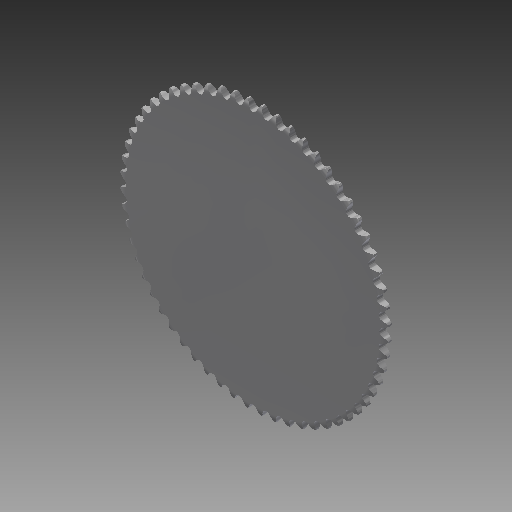
# Autodesk Inventor part: Roller Chain Sprocket2
Saved by Autodesk Inventor 2018.2 (Build 222227000, 227)
## iProperties
Created: 2018-02-09
Part Number: Roller Chain Sprocket2
Material: Steel
Document SubType Name: Modeling
Designer: steele
Density: 1 g/cm^3
Appearance: Steel
CustomPartVersion: 1
Author: steele
Autodesk Inventor part; units mm, degrees
ref_plane "YZ Plane" through (0, 0, 0) normal (1, 0, 0) x (0, 1, 0)
ref_plane "XZ Plane" through (0, 0, 0) normal (0, 1, 0) x (-1, 0, 0)
ref_plane "XY Plane" through (0, 0, 0) normal (0, 0, 1) x (1, 0, 0)
sketch "Theoretical Tooth Profile" plane through (0, 0, 0) normal (0, 0, 1) x (1, 0, 0)
  circle A0 centre (0, 0) radius 90.9986 construction
  line L0 (0, 0) -> (0, 90.9986) construction
  line L1 (0, 0) -> (9.5119, 90.5001) construction
  circle A1 centre (0, 0) radius 93.7314
  arc A2 (-2.096, 89.4758) -> (2.096, 89.4758) centre (0, 90.9986) ccw
  line L2 (0, 90.9986) -> (9.5119, 90.5001) construction
  line L3 (0, 90.9986) -> (3.2878, 93.3874) construction
  line L4 (3.2878, 93.3874) -> (-3.0069, 91.2281) construction
  arc A3 (4.3573, 93.6301) -> (3.2534, 91.9467) centre (7.1023, 90.6264) ccw
  arc A4 (-3.2534, 91.9467) -> (-4.3573, 93.6301) centre (-7.1023, 90.6264) ccw
  line L5 (-7.1023, 90.6264) -> (-3.2534, 91.9467) construction
  arc A5 (-3.0069, 91.2281) -> (-2.096, 89.4758) centre (3.2878, 93.3874) ccw
  line L6 (-3.0069, 91.2281) -> (-3.2534, 91.9467)
  arc A6 (2.096, 89.4758) -> (3.0069, 91.2281) centre (-3.2878, 93.3874) ccw
  line L7 (3.2534, 91.9467) -> (3.0069, 91.2281)
  line L8 (0, 0) -> (4.9055, 93.603) construction
  point P0 (4.756, 90.7494)
  dimension "d0" = 181.9973
  dimension "d2" = 6
  dimension "d3" = 2.5908
  dimension "d10" = 126
  dimension "d11" = 17.067
  dimension "d12" = 4.064
  dimension "d13" = 6.6548
  dimension "d14" = 7.112
  dimension "d23" = 2.8575
  constraints: 18 end point, 15 point on circle, 7 centre point, 3 coincident, 3 point on line, 3 symmetric about line, 3 tangent, 1 equal radius, 1 midpoint, 1 parallel, 1 vertical, 1 other
  measures "d0" diameter of A0
  measures "d2" angle of L1 L0
  measures "d3" radius of A2
  measures "d10" angle of L3 L0
  measures "d11" angle of L4 L3
  measures "d12" distance of L2.start L3.end
  measures "d13" distance of L3.end L4.end
  measures "d14" distance of A3.centre L0.end
  measures "d23" distance from line of L8.end L2
sketch "Tooth Profile" plane through (0, 0, 0) normal (0, 0, 1) x (1, 0, 0)
  circle A0 centre (0, 0) radius 93.7314 projected
  line L0 (0, 0) -> (0, 90.9986) construction
  line L1 (0, 90.9986) -> (2.4227, 90.0807) construction
  arc A1 (-2.4227, 90.0807) -> (2.4227, 90.0807) centre (0, 90.9986) ccw
  line L2 (-2.4227, 90.0807) -> (0, 90.9986) construction
  arc A2 (-2.4227, 90.0807) -> (-3.9883, 93.6465) centre (-37.7664, 76.6902) ccw
  arc A3 (3.9883, 93.6465) -> (2.4227, 90.0807) centre (37.7664, 76.6902) ccw
  dimension "d44" = 138.5
  dimension "d45" = 2.5908
  dimension "d46" = 37.7952
  constraints: 8 point on circle, 7 end point, 3 centre point, 2 tangent, 1 coincident, 1 equal radius, 1 symmetric about line, 1 vertical
  measures "d44" angle of L1 L2
  measures "d45" radius of A1
  measures "d46" radius of A3
sketch "Section Profile" plane through (0, 0, 0) normal (1, 0, 0) x (0, 1, 0)
  line L0 (93.7314, 0) -> (-93.7314, 0) projected
  line L1 (85.3494, 2.2967) -> (-85.3494, 2.2967)
  line L2 (-85.3494, 2.2967) -> (-85.3494, -2.2967)
  line L3 (-85.3494, -2.2967) -> (85.3494, -2.2967)
  line L4 (85.3494, -2.2967) -> (85.3494, 2.2967)
  line L5 (85.3494, 2.2967) -> (93.7314, 2.2967) construction
  line L6 (93.7314, 2.2967) -> (93.7314, -2.2967) construction
  line L7 (93.7314, -2.2967) -> (85.3494, -2.2967) construction
  line L8 (85.3494, -2.2967) -> (85.3494, 2.2967)
  arc A0 (93.7314, 1.106) -> (88.9677, 2.2967) centre (88.9677, -7.8284) ccw
  arc A1 (88.9677, -2.2967) -> (93.7314, -1.106) centre (88.9677, 7.8284) ccw
  line L9 (88.9677, 2.2967) -> (0, 2.2967)
  line L10 (0, 2.2967) -> (0, -2.2967)
  line L11 (0, -2.2967) -> (88.9677, -2.2967)
  line L12 (0, 2.2967) -> (0, -2.2967)
  line L13 (93.7314, 1.106) -> (93.7314, -1.106)
  point P0 (0, 0)
  point P1 (0, 0)
  dimension "d30" = 4.5933
  dimension "d31" = 170.6988
  dimension "d32" = 4.5933
  dimension "d33" = 1.1906
  dimension "d34" = 10.1251
  dimension "d43" = 2.2967
  constraints: 26 end point, 7 midpoint, 5 perpendicular, 4 parallel, 4 point on circle, 3 point on line, 3 symmetric about line, 2 centre point, 2 horizontal, 2 tangent, 1 collinear, 1 other
  measures "d30" distance between parallel lines of L7 L5
  measures "d31" distance between parallel lines of L2 L4
  measures "d32" distance between parallel lines of L3 L1
  measures "d33" distance from line of L13.start L5
  measures "d34" radius of A0
  measures "d43" distance between parallel lines of L3 L0
revolve "Shroud" add sketch "Section Profile" angle 360 about axis through (0, 0, 2.2967) along (0, 0, -1) contours L10 L3 L2 L0 | L0 L2 L1 L10
revolve "Strand" add sketch "Section Profile" angle 360 about axis through (0, 0, 2.2967) along (0, 0, -1) contours L13 A1 L11 L4 L0 | L0 L4 L9 A0 L13 | L4 L3 L10 L0 | L0 L10 L1 L4
pattern_of_one "Strand Pattern"
extrude "Theoretical Tooth" cut sketch "Theoretical Tooth Profile" along normal through all both and the other way through all contours A3 L7 A6 A2 A5 L6 A4 A1 picked at (0.4843, 91.2592)
extrude "Tooth" [suppressed]
pattern_circular "Tooth Pattern" count 60 over 360 about axis through (0, 0, -10) along (0, 0, 1) of "Theoretical Tooth"
ref_plane "Timing Plane" through (0, 90.9986, 0) normal (1, 0, 0) x (0, 1, 0)
equation "\"d3\" = 0.5 * da_Dr + da_SC"
equation "\"d12\" = 0.8 * da_Dr"
equation "\"d13\" = 1.3 * da_Dr + da_SC"
equation "\"d14\" = 1.4 * da_Dr"
equation "\"d23\" = da_Ha"
equation "\"d44\" = da_Alfa"
equation "\"d45\" = da_Ri"
equation "\"d46\" = da_Re"
equation "\"d30\" = da_Bf"
equation "\"d31\" = da_Ds"
equation "\"d32\" = da_Bs"
equation "\"d33\" = da_Ba"
equation "\"d34\" = da_Rx"
equation "\"d40\" = da_pt"
equation "\"form_type\" = 0"
equation "\"da_p\" = 9.525"
equation "\"da_Dr\" = 5.08"
equation "\"da_SC\" = 0.0508"
equation "\"da_Ha\" = 2.8575"
equation "\"da_pt\" = 10.1346"
equation "\"da_Bf\" = 4.59334"
equation "\"da_Ba\" = 1.19063"
equation "\"da_Rx\" = 10.12508"
equation "\"da_Ra\" = 0.381"
equation "\"da_Bs\" = 4.59334"
equation "\"da_Ds\" = 170.69883"
equation "\"da_Re\" = 37.7952"
equation "\"da_Ri\" = 2.5908"
equation "\"da_Alfa\" = 138.5deg"
body "Solid1"
